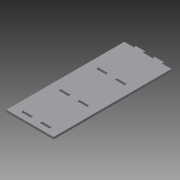
# Autodesk Inventor part: tapa laterales
Saved by Autodesk Inventor 2015 (Build 190159000, 159)
## iProperties
Created: 2016-01-26
Part Number: tapa laterales
Material: Generic
Document SubType Name: Modeling
Designer: iberopuebla
Density: 1 g/cm^3
Appearance: Default
Author: iberopuebla
Autodesk Inventor part; units mm, degrees
ref_plane "YZ Plane" through (0, 0, 0) normal (1, 0, 0) x (0, 1, 0)
ref_plane "XZ Plane" through (0, 0, 0) normal (0, 1, 0) x (-1, 0, 0)
ref_plane "XY Plane" through (0, 0, 0) normal (0, 0, 1) x (1, 0, 0)
sketch "Sketch1" plane through (0, 0, 0) normal (0, 0, 1) x (1, 0, 0)
  line L0 (0, 0) -> (400, 0)
  line L1 (400, 0) -> (400, 1000)
  line L2 (0, 1000) -> (0, 0)
  line L3 (80, 1002.5) -> (80, 1018)
  line L4 (160, 1002.5) -> (160, 1018)
  line L5 (240, 1002.5) -> (240, 1018)
  line L6 (320, 1002.5) -> (320, 1018)
  line L7 (80, 1018) -> (160, 1018)
  line L8 (240, 1018) -> (320, 1018)
  line L9 (400, 1000) -> (322.5, 1000)
  line L10 (237.5, 1000) -> (162.5, 1000)
  arc A0 (77.5, 1000) -> (80, 1002.5) centre (80, 1000) ccw
  arc A1 (160, 1002.5) -> (162.5, 1000) centre (160, 1000) ccw
  arc A2 (237.5, 1000) -> (240, 1002.5) centre (240, 1000) ccw
  arc A3 (320, 1002.5) -> (322.5, 1000) centre (320, 1000) ccw
  line L11 (0, 1000) -> (77.5, 1000)
  line L12 (80, 697.5) -> (80, 684.5)
  line L13 (160, 697.5) -> (160, 684.5)
  line L14 (240, 697.5) -> (240, 684.5)
  line L15 (320, 697.5) -> (320, 684.5)
  line L16 (82.5, 682) -> (157.5, 682)
  line L17 (242.5, 682) -> (317.5, 682)
  line L18 (82.5, 700) -> (157.5, 700)
  line L19 (242.5, 700) -> (317.5, 700)
  line L20 (80, 379.5) -> (80, 366.5)
  line L21 (80, 61.5003) -> (80, 48.5)
  line L22 (160, 379.5003) -> (160, 366.5)
  line L23 (160, 61.5003) -> (160, 48.5)
  line L24 (240, 379.5) -> (240, 366.5)
  line L25 (240, 61.5) -> (240, 48.5)
  line L26 (320, 379.5) -> (320, 366.4997)
  line L27 (320, 61.5003) -> (320, 48.5)
  line L28 (82.5, 382) -> (157.4609, 382)
  line L29 (82.5, 364) -> (157.5, 364)
  line L30 (242.5, 364) -> (317.4609, 364)
  line L31 (82.5, 64) -> (157.4609, 64)
  line L32 (242.5, 64) -> (317.4609, 64)
  line L33 (82.5, 46) -> (157.5, 46)
  line L34 (242.5, 46) -> (317.5, 46)
  arc A4 (82.5, 700) -> (80, 697.5) centre (80, 700) ccw
  arc A5 (160, 697.5) -> (157.5, 700) centre (160, 700) ccw
  arc A6 (157.5, 682) -> (160, 684.5) centre (160, 682) ccw
  arc A7 (80, 684.5) -> (82.5, 682) centre (80, 682) ccw
  arc A8 (242.5, 700) -> (240, 697.5) centre (240, 700) ccw
  arc A9 (240, 684.5) -> (242.5, 682) centre (240, 682) ccw
  arc A10 (320, 697.5) -> (317.5, 700) centre (320, 700) ccw
  arc A11 (317.5, 682) -> (320, 684.5) centre (320, 682) ccw
  arc A12 (320, 379.5) -> (317.5, 382) centre (320, 382) ccw
  arc A13 (317.4609, 364) -> (320, 366.4997) centre (319.9609, 364) ccw
  arc A14 (242.5, 382) -> (240, 379.5) centre (240, 382) ccw
  arc A15 (240, 366.5) -> (242.5, 364) centre (240, 364) ccw
  arc A16 (157.5, 364) -> (160, 366.5) centre (160, 364) ccw
  arc A17 (160, 379.5003) -> (157.4609, 382) centre (159.9609, 382) ccw
  arc A18 (82.5, 382) -> (80, 379.5) centre (80, 382) ccw
  arc A19 (80, 366.5) -> (82.5, 364) centre (80, 364) ccw
  arc A20 (82.5, 64) -> (80, 61.5003) centre (80, 64.0003) ccw
  arc A21 (160, 61.5003) -> (157.4609, 64) centre (159.9609, 64) ccw
  arc A22 (157.5, 46) -> (160, 48.5) centre (160, 46) ccw
  arc A23 (80, 48.5) -> (82.5, 46) centre (80, 46) ccw
  arc A24 (242.5, 64) -> (240, 61.5) centre (240, 64) ccw
  arc A25 (320, 61.5003) -> (317.4609, 64) centre (319.9609, 64) ccw
  arc A26 (317.5, 46) -> (320, 48.5) centre (320, 46) ccw
  arc A27 (240, 48.5) -> (242.5, 46) centre (240, 46) ccw
  line L35 (242.5, 382) -> (317.5, 382)
  dimension "d1" = 1000
  dimension "d4" = 80
  dimension "d5" = 80
  dimension "d6" = 80
  dimension "d7" = 400
  dimension "d9" = 5
  dimension "d10" = 5
  dimension "d11" = 5
  dimension "d12" = 5
  dimension "d19" = 80
  dimension "d20" = 80
  dimension "d21" = 80
  dimension "d22" = 80
  dimension "d23" = 18
  dimension "d24" = 18
  dimension "d31" = 80
  dimension "d33" = 80
  dimension "d34" = 80
  dimension "d38" = 18
  dimension "d41" = 18
  dimension "d42" = 18
  dimension "d43" = 80
  dimension "d44" = 80
  dimension "d45" = 80
  dimension "d46" = 80
  dimension "d47" = 5
  dimension "d48" = 5
  dimension "d49" = 5
  dimension "d50" = 5
  dimension "d51" = 5
  dimension "d52" = 5
  dimension "d53" = 5
  dimension "d54" = 5
  dimension "d55" = 5
  dimension "d56" = 5
  dimension "d57" = 5
  dimension "d58" = 5
  dimension "d59" = 5
  dimension "d60" = 5
  dimension "d61" = 5
  dimension "d62" = 5
  dimension "d63" = 5
  dimension "d64" = 5
  dimension "d65" = 5
  dimension "d66" = 5
  dimension "d67" = 5
  dimension "d68" = 5
  dimension "d69" = 5
  dimension "d70" = 5
  dimension "d71" = 80
  dimension "d72" = 18
  constraints: 72 end point, 56 point on circle, 28 centre point, 24 perpendicular, 9 horizontal, 3 parallel, 1 vertical, 24 other
  measures "d1" distance of L2.start L0.start
  measures "d4" distance between parallel lines of L4 L3
  measures "d5" distance between parallel lines of L4 L5
  measures "d6" distance between parallel lines of L6 L5
  measures "d7" distance between parallel lines of L1 L2
  measures "d9" diameter of A0
  measures "d10" diameter of A1
  measures "d11" diameter of A2
  measures "d12" diameter of A3
  measures "d19" distance between parallel lines of L2 L12
  measures "d20" distance between parallel lines of L13 L12
  measures "d21" distance between parallel lines of L14 L13
  measures "d22" distance between parallel lines of L15 L14
  measures "d23" distance between parallel lines of L16 L18
  measures "d24" distance between parallel lines of L17 L19
  measures "d31" distance of L20.start L22.start
  measures "d33" distance between parallel lines of L24 L22
  measures "d34" distance between parallel lines of L2 L20
  measures "d38" distance between parallel lines of L28 L29
  measures "d41" distance between parallel lines of L32 L34
  measures "d42" distance between parallel lines of L31 L33
  measures "d43" distance between parallel lines of L2 L21
  measures "d44" distance of L21.start L23.start
  measures "d45" distance between parallel lines of L25 L23
  measures "d46" distance of L25.start L27.start
  measures "d47" diameter of A4
  measures "d48" diameter of A5
  measures "d49" diameter of A6
  measures "d50" diameter of A7
  measures "d51" diameter of A8
  measures "d52" diameter of A9
  measures "d53" diameter of A10
  measures "d54" diameter of A11
  measures "d55" diameter of A12
  measures "d56" diameter of A13
  measures "d57" diameter of A14
  measures "d58" diameter of A15
  measures "d59" diameter of A16
  measures "d60" diameter of A17
  measures "d61" diameter of A18
  measures "d62" diameter of A19
  measures "d63" diameter of A20
  measures "d64" diameter of A21
  measures "d65" diameter of A22
  measures "d66" diameter of A23
  measures "d67" diameter of A24
  measures "d68" diameter of A25
  measures "d69" diameter of A26
  measures "d70" diameter of A27
  measures "d71" distance between parallel lines of L26 L24
  measures "d72" distance between parallel lines of L30 L35
extrude "Extrusion1" add sketch "Sketch1" along normal blind 18
body "Solid1"
